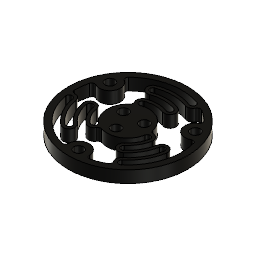
Spring (parametric) (Autodesk Fusion 360 design; units mm, degrees)
Autodesk Fusion 360 part; units mm, degrees
sketch "Base" plane through (0, 0, 0) normal (0, 0, 1) x (1, 0, 0)
  circle A0 centre (0, 0) radius 20
  line L0 (0, 0) -> (0, 20) construction
  line L1 (0, 0) -> (-6.8404, 18.7939) construction
  line L2 (0, 0) -> (6.8404, 18.7939) construction
  arc A1 (3.2492, 8.9271) -> (-3.2492, 8.9271) centre (0, 0) ccw
  circle A2 centre (0, 0) radius 18
  circle A3 centre (0, 0) radius 7
  arc A4 (4.2753, 11.7462) -> (-4.2753, 11.7462) centre (0, 0) ccw
  arc A5 (5.3013, 14.5652) -> (-5.3013, 14.5652) centre (0, 0) ccw
  arc A6 (-5.3013, 14.5652) -> (-4.2753, 11.7462) centre (-4.7883, 13.1557) ccw
  arc A7 (3.2492, 8.9271) -> (4.2753, 11.7462) centre (3.7622, 10.3366) ccw
  arc A8 (5.3013, 14.5652) -> (6.3274, 17.3843) centre (5.8143, 15.9748) ccw
  arc A9 (-3.2492, 8.9271) -> (-2.2231, 6.108) centre (-2.7362, 7.5175) ccw
  line L3 (0, 0) -> (17.3205, 10) construction
  circle A10 centre (14.2894, 8.25) radius 3.5
  circle A11 centre (0, 0) radius 4 construction
  point P0 (6.1564, 16.9145)
  point P1 (-2.3941, 6.5778)
  point P2 (3.4641, 2)
  dimension "d6" = 40
  dimension "d7" = 40
  dimension "d9" = -2
  dimension "d10" = 14
  dimension "d11" = 0.5
  dimension "d13" = 7
  dimension "d15" = 8
  dimension "d34" = 40
  dimension "d35" = 0.5
  constraint coincident A0.centre L0.start
  constraint coincident A0 L0.end
  constraint vertical L0
  constraint coincident A0 L1.end
  constraint symmetric L0 A0.centre L1.start
  constraint symmetric L0 L1.end L2.end
  constraint coincident L2 A1.start
  constraint coincident L1 A1.end
  constraint coincident L2 A4.start
  constraint coincident L1 A4.end
  constraint coincident L2 A5.start
  constraint coincident L1 A5.end
  constraint coincident L2 A8.end
  constraint coincident L1 A9.end
  constraint equal A6 A8
  constraint equal A6 A7
  constraint equal A7 A9
  constraint tangent A5 A6
  constraint tangent A4 A7
  constraint tangent A5 A8
  constraint tangent A1 A9
  constraint coincident A2 P0
  constraint coincident L2 P0
  constraint coincident L1 P1
  constraint coincident A3 P1
  constraint coincident L3 A10.centre
  constraint coincident A0 L3.end
  constraint tangent A0 A10
  constraint coincident A11 P2
  constraint coincident L3 P2
  measures "d6" diameter of A0
  measures "d7" angle of L1 L2
  measures "d10" diameter of A3
  measures "d11" distance of A9.end P1
  measures "d13" diameter of A10
  measures "d15" diameter of A11
  measures "d34" angle of L2 L3
  measures "d35" distance of A8.end P0
extrude "Extrude1" add sketch "Base" along normal blind 4 contours A2 A10 | A0 | A3 picked at (16.1463, 9.3221) makes body 1 at (19.9006, 1.9914, 2.6667) makes body 2 at (6.9913, -0.3489, 1.3333)
ref_plane "WorkPlane1" through (0, 10, 0) normal (1, 0, 0) x (0, 1, 0)
sketch "Spring Blade" plane through (0, 0, 0) normal (1, 0, 0) x (0, 1, 0)
  line L0 (12.5, 0) -> (11.7462, 0)
  line L1 (12.5, 0) -> (12.5, 4) construction
  line L2 (12, 4) -> (13, 4)
  line L3 (13, 4) -> (13, 0)
  line L4 (13, 0) -> (12, 0)
  line L5 (12, 0) -> (12, 4)
  line L6 (12, 4) -> (13, 0) construction
  line L7 (13, 4) -> (12, 0) construction
  point P0 (12.5, 2)
  dimension "d36" = 4
  dimension "d37" = 1
  constraint coincident L0.start L1.start
  constraint perpendicular L0 L1
  constraint horizontal L2
  constraint perpendicular L2 L3
  constraint parallel L2 L4
  constraint parallel L3 L5
  constraint coincident L6 P0
  constraint coincident L7 P0
  constraint midpoint L1 P0
  constraint midpoint L0.start L4
  measures "d36" distance of L0.start L1.end
  measures "d37" distance of L3 L5
sweep "Sweep2" add profiles "Spring Blade" path "Base" along A9 A1 A7 A4 A6 A5 A8 section 1 bodies 1 2
extrude "Extrude3" add sketch "Base" along normal up to surface (4 mm away) contours A2 A10 picked at (14.1256, 8.1554) bodies 1
pattern_circular "C-Pattern2" count 3 over 360 about axis through (0, 0, 1.75) along (0, 0, 1) of "Sweep2", "Extrude3"
hole "Hole1" at (3.4641, 2, 0) at (14.2894, 8.25, 0) direction (0, 0, 1) diameter 3.2 end through all bodies 1
pattern_circular "C-Pattern3" count 3 over 360 about axis through (0, 0, 1.75) along (0, 0, 1) of "Hole1"
fillet "Fillet1" radius 1 12 edges at (7.7989, 16.2227, 2) (-13.6815, 11.6968, 2) (-16.9705, 6.0002, 2) (13.6815, 11.6968, 2) (16.9705, 6.0002, 2) (3.289, -17.697, 2) (10.1498, -14.8654, 2) (-17.9488, -1.3573, 2) (-3.289, -17.697, 2) (-3.8423, 5.8512, 2) (-3.1462, -6.2531, 2) (6.9885, 0.4019, 2) on bodies 1
equation "o_diam = 40 mm"
equation "spring_n = 3"
equation "spring_angle = 40 deg"
equation "spring_blade = 1 mm"
equation "spring_height = 4 mm"
equation "d6 = o_diam"
equation "d7 = spring_angle"
equation "d9 = -ceil(spring_blade * 1.5)"
equation "d10 = central_hub"
equation "d11 = spring_blade / 2"
equation "d15 = central_hub - 6 mm"
equation "d18 = spring_height"
equation "central_hub = 14 mm"
equation "d34 = ( ( 360 deg - ( spring_n * spring_angle ) ) / spring_n ) / 2"
equation "d35 = spring_blade / 2"
equation "d36 = spring_height"
equation "d37 = spring_blade"
equation "d48 = spring_n"
equation "d50 = spring_n"
